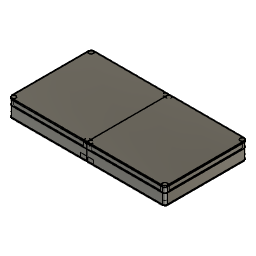
v1.3 (Autodesk Fusion 360 design; units mm, degrees)
Autodesk Fusion 360 part; units mm, degrees
(part 1 of 2)
sketch "Sketch1" plane through (0, 0, 0) normal (0, 0, 1) x (1, 0, 0)
  line L0 (192.147805, -6) -> (205.147805, -6) construction
  line L1 (192.147805, -6) -> (179.147805, -6) construction
  circle A0 centre (179.146093, -187.967124) radius 2
  circle A1 centre (13.147805, -188) radius 2
  line L2 (13.147805, -6) -> (13.147805, -16) construction
  circle A2 centre (205.147805, -16) radius 2
  line L3 (13.147805, -198) -> (13.147805, -188) construction
  line L4 (384.147805, -198) -> (371.147805, -198) construction
  line L5 (179.147805, -26) -> (13.147805, -26)
  line L6 (192.147805, -197.967124) -> (179.147805, -197.967124) construction
  line L7 (384.147805, -6) -> (371.147805, -6) construction
  line L8 (179.147805, -6) -> (179.147805, -26) construction
  line L9 (192.147805, -197.967124) -> (0.147805, -198)
  line L10 (205.147805, -197.967124) -> (205.147805, -187.967124) construction
  line L11 (0.147805, -198) -> (0.147805, -6)
  circle A3 centre (179.147805, -16) radius 2
  line L12 (384.147805, -198) -> (384.147805, -6)
  line L13 (371.147805, -26) -> (205.147805, -26)
  line L14 (371.147805, -198) -> (371.147805, -188) construction
  line L15 (205.147805, -26) -> (205.147805, -177.967124)
  line L16 (13.147805, -178) -> (179.147805, -178)
  line L17 (0.147805, -198) -> (13.147805, -198) construction
  line L18 (205.147805, -197.967124) -> (205.147805, -177.967124) construction
  circle A4 centre (205.147805, -187.967124) radius 2
  line L19 (0.147805, -198) -> (13.147805, -198) construction
  line L20 (371.147805, -6) -> (371.147805, -16) construction
  line L21 (192.147805, -6) -> (179.147805, -6) construction
  circle A5 centre (13.147805, -16) radius 2
  circle A6 centre (371.147805, -16) radius 2
  line L22 (192.147805, -6) -> (192.147805, -197.967124) construction
  line L23 (179.147805, -6) -> (179.147805, -16) construction
  line L24 (371.147805, -6) -> (371.147805, -26) construction
  line L25 (205.147805, -6) -> (205.147805, -16) construction
  line L26 (13.147805, -26) -> (13.147805, -178)
  line L27 (384.147805, -6) -> (0.147805, -6)
  line L28 (179.147805, -197.967124) -> (179.146093, -187.967124) construction
  line L29 (13.147805, -198) -> (13.147805, -178) construction
  line L30 (0.147805, -6) -> (13.147805, -6) construction
  line L31 (179.147805, -178) -> (179.147805, -26)
  line L32 (192.147805, -197.967124) -> (205.147805, -197.967124) construction
  line L33 (0.147805, -6) -> (0.147805, -198)
  line L34 (205.147805, -177.967124) -> (371.147805, -177.967124)
  circle A7 centre (371.147805, -188) radius 2
  line L35 (384.147805, -6) -> (371.147805, -6) construction
  line L36 (371.147805, -177.967124) -> (371.147805, -26)
  line L37 (0.147805, -198) -> (384.147805, -198)
  line L38 (192.147805, -197.967124) -> (205.147805, -197.967124) construction
  line L39 (384.147805, -6) -> (384.147805, 12.021307) construction
  line L40 (0.147805, -6) -> (-9.044583, 3.192388) construction
  line L41 (0.147805, -6) -> (15, -6) construction
  circle A8 centre (-4.448389, -1.403806) radius 6.5
  line L42 (0.147805, -198) -> (-9.044583, -207.192388) construction
  line L43 (384.147805, -198) -> (393.340193, -207.192388) construction
  line L44 (384.147805, -198) -> (399, -198) construction
  line L45 (384.147805, -6) -> (393.340193, 3.192388) construction
  line L46 (384.147805, -6) -> (399, -6) construction
  circle A9 centre (388.743999, -1.403806) radius 6.5
  circle A10 centre (388.743999, -202.596194) radius 6.5
  circle A11 centre (-4.448389, -202.596194) radius 6.5
  line L47 (-10.930518, -1.885465) -> (-10.948389, -202.595615)
  line L48 (-4.448389, -209.096194) -> (388.743999, -209.096194)
  line L49 (395.243999, -202.596194) -> (395.243999, -1.403806)
  line L50 (-4.448389, 5.096194) -> (388.743999, 5.096194)
  line L51 (388.743999, -202.596194) -> (395.243999, -202.596194) construction
  line L52 (-4.448389, -1.403806) -> (-4.448389, 5.096194) construction
  point P0 (13, -13)
  dimension "d13" = 192
  dimension "d14" = 192
  dimension "d15" = 384
  dimension "d16" = 384
  dimension "d20" = 13
  dimension "d21" = 10
  dimension "d22" = 4
  dimension "d23" = 13
  dimension "d24" = 10
  dimension "d25" = 13
  dimension "d26" = 10
  dimension "d27" = 13
  dimension "d28" = 10
  dimension "d29" = 13
  dimension "d30" = 10
  dimension "d31" = 13
  dimension "d32" = 10
  dimension "d33" = 13
  dimension "d34" = 10
  dimension "d35" = 13
  dimension "d36" = 10
  dimension "d37" = 4
  dimension "d38" = 4
  dimension "d39" = 4
  dimension "d40" = 4
  dimension "d41" = 4
  dimension "d42" = 4
  dimension "d43" = 4
  dimension "d44" = 13
  dimension "d45" = 20
  dimension "d46" = 13
  dimension "d47" = 20
  dimension "d48" = 13
  dimension "d49" = 20
  dimension "d50" = 13
  dimension "d51" = 20
  dimension "d69" = 135
  dimension "d70" = 13
  dimension "d71" = 13
  dimension "d72" = 45
  dimension "d73" = 13
  dimension "d74" = 13
  dimension "d75" = 45
  dimension "d104" = 135
  constraint perpendicular L11 L30
  constraint perpendicular L2 L30
  constraint perpendicular L7 L12
  constraint perpendicular L7 L20
  constraint perpendicular L4 L12
  constraint perpendicular L14 L37
  constraint perpendicular L19 L33
  constraint perpendicular L3 L19
  constraint perpendicular L22 L37
  constraint perpendicular L6 L22
  constraint perpendicular L9 L28
  constraint perpendicular L21 L22
  constraint perpendicular L21 L23
  constraint perpendicular L0 L22
  constraint perpendicular L25 L27
  constraint perpendicular L22 L32
  constraint perpendicular L10 L32
  constraint perpendicular L11 L17
  constraint perpendicular L17 L29
  constraint perpendicular L1 L22
  constraint perpendicular L1 L8
  constraint horizontal L16
  constraint vertical L31
  constraint horizontal L5
  constraint vertical L26
  constraint perpendicular L22 L38
  constraint perpendicular L18 L38
  constraint perpendicular L20 L35
  constraint perpendicular L24 L35
  constraint horizontal L34
  constraint vertical L36
  constraint horizontal L13
  constraint vertical L15
  constraint perpendicular L7 L39
  constraint horizontal L41
  constraint horizontal L44
  constraint horizontal L46
  constraint tangent A11 L47
  constraint tangent A10 L48
  constraint tangent A9 L49
  constraint perpendicular L46 L49
  constraint tangent A9 L50
  constraint perpendicular L49 L50
  constraint tangent A11 L48
  constraint parallel L48 L51
  constraint vertical L52
  measures "d22" diameter of A5
  measures "d37" diameter of A1
  measures "d38" diameter of A3
  measures "d39" diameter of A0
  measures "d40" diameter of A2
  measures "d41" diameter of A4
  measures "d42" diameter of A7
  measures "d43" diameter of A6
  measures "d69" angle of L40 L41
  measures "d72" angle of L43 L44
  measures "d75" angle of L45 L46
  measures "d104" angle of L37 L42
extrude "Extrude1" add sketch "Sketch1" along normal blind 2 contours L11 L33 A8 A11 L47 | L11 L12 L27 L33 L37 | L37 A10 A11 L48 | A11 | L27 A8 A9 L50 | A8 | L12 A9 A10 L49 | A10 | A9 picked at (-4.706637, -133.373076) picked at (187.814472, -127.322375) picked at (255.526246, -202.702251) picked at (-2.560006, -204.6862) picked at (255.526246, -1.297749) picked at (-3.056002, -1.357586) picked at (389.062427, -70.631992) picked at (386.660446, -202.382039) picked at (392.395412, 0.127516) makes body 1
sketch "Sketch3" plane through (0, 0, 2) normal (0, 0, 1) x (-1, 0, 0)
  arc A0 (-395.243999, 1.403816) -> (-388.743999, -5.096194) centre (-388.743999, 1.403806) ccw
  line L0 (-388.743999, -5.096194) -> (4.448389, -5.096194)
  arc A1 (4.448389, -5.096194) -> (10.930518, 1.885465) centre (4.448389, 1.403806) ccw
  circle A2 centre (4.448389, 1.403806) radius 5.5
  circle A3 centre (4.448389, 202.596194) radius 5.5
  circle A4 centre (-388.743999, 202.596194) radius 5.5
  circle A5 centre (-388.743999, 1.403806) radius 5.5
  line L1 (-388.743999, -4.096194) -> (4.448389, -4.096194)
  line L2 (9.948389, 1.403806) -> (9.948389, 202.596194)
  line L3 (3.313779, 207.977891) -> (-388.74234, 208.096194)
  line L4 (-394.243998, 202.59619) -> (-394.243999, 1.403806)
  line L5 (-192.147805, -4.096194) -> (-192.714281, 208.037042) construction
  circle A6 centre (-187.161139, 0.903806) radius 5
  circle A7 centre (-197.161175, 0.903806) radius 5
  circle A8 centre (-187.700907, 203.035529) radius 5
  circle A9 centre (-197.70095, 203.038547) radius 5
  line L6 (-182.700907, 203.035529) -> (-182.700907, 208.034021)
  line L7 (-202.700834, 203.072636) -> (-202.666966, 208.040046)
  line L8 (-187.161145, 5.903806) -> (-197.161175, 5.903806)
  line L9 (-202.161175, 0.903806) -> (-202.161175, -4.096194)
  line L10 (-182.161139, 0.903806) -> (-182.161139, -4.096194)
  line L11 (-383.661991, 197.999703) -> (-384.000006, 6)
  line L12 (0.338009, 197.999703) -> (-383.661991, 197.999703)
  line L13 (-0.000006, 6) -> (0.338009, 197.999703)
  line L14 (-384.000006, 6) -> (-0.000006, 6)
  line L15 (4.448389, 6.903806) -> (9.948389, 6.903806)
  line L16 (-1.051611, 1.403806) -> (-1.051611, -4.096194)
  line L17 (-383.243999, 1.403806) -> (-383.243999, -4.096194)
  line L18 (-388.743999, 6.903806) -> (-394.243999, 6.903806)
  line L19 (-388.743999, 197.096194) -> (-394.243998, 197.096194)
  line L20 (-383.243999, 202.596194) -> (-383.243999, 208.094535)
  line L21 (4.448389, 197.096194) -> (9.948389, 197.096194)
  line L22 (-1.051611, 202.596194) -> (-1.051611, 207.979208)
  circle A10 centre (-13.147805, 188) radius 2
  circle A11 centre (-179.146093, 187.967124) radius 2
  circle A12 centre (-205.147805, 16) radius 2
  circle A13 centre (-179.147805, 16) radius 2
  circle A14 centre (-205.147805, 187.967124) radius 2
  circle A15 centre (-13.147805, 16) radius 2
  circle A16 centre (-371.147805, 16) radius 2
  line L23 (-179.147805, 26) -> (-179.147805, 178)
  line L24 (-179.147805, 178) -> (-13.147805, 178)
  line L25 (-13.147805, 178) -> (-13.147805, 26)
  line L26 (-13.147805, 26) -> (-179.147805, 26)
  line L27 (-371.147805, 26) -> (-371.147805, 177.967124)
  line L28 (-371.147805, 177.967124) -> (-205.147805, 177.967124)
  line L29 (-205.147805, 177.967124) -> (-205.147805, 26)
  line L30 (-205.147805, 26) -> (-371.147805, 26)
  circle A17 centre (-371.147805, 188) radius 2
  line L31 (10.930518, 1.885465) -> (10.948389, 202.595615)
  arc A18 (10.948389, 202.595615) -> (4.448389, 209.096194) centre (4.448389, 202.596194) ccw
  line L32 (4.448389, 209.096194) -> (-388.743999, 209.096194)
  arc A19 (-388.743999, 209.096194) -> (-395.243999, 202.596194) centre (-388.743999, 202.596194) ccw
  line L33 (-395.243999, 202.596194) -> (-395.243999, 1.403816)
  line L34 (-187.700907, 198.035529) -> (-197.702459, 198.038547)
  dimension "d76" = 11
  dimension "d77" = 11
  dimension "d78" = 11
  dimension "d79" = 11
  dimension "d80" = 5
  dimension "d81" = 5
  dimension "d82" = 5
  dimension "d83" = 5
  dimension "d85" = 192
  dimension "d87" = 384
  constraint concentric A1 A2
  constraint concentric A0 A5
  constraint tangent A2 L1
  constraint parallel L0 L1
  constraint tangent A3 L2
  constraint tangent A4 L3
  constraint tangent A5 L4
  constraint tangent L1 A6
  constraint tangent L5 A6
  constraint tangent L5 A7
  constraint tangent L1 A7
  constraint tangent L5 A8
  constraint tangent L3 A8
  constraint tangent L5 A9
  constraint tangent L3 A9
  constraint tangent A8 L6
  constraint vertical L6
  constraint tangent A9 L7
  constraint tangent A7 L8
  constraint horizontal L8
  constraint tangent A7 L9
  constraint perpendicular L1 L9
  constraint tangent A6 L10
  constraint perpendicular L1 L10
  constraint tangent A2 L15
  constraint horizontal L15
  constraint tangent A2 L16
  constraint perpendicular L1 L16
  constraint tangent A5 L17
  constraint perpendicular L1 L17
  constraint tangent A5 L18
  constraint perpendicular L4 L18
  constraint tangent A4 L19
  constraint perpendicular L4 L19
  constraint tangent A4 L20
  constraint vertical L20
  constraint tangent A3 L21
  constraint horizontal L21
  constraint tangent A3 L22
  constraint vertical L22
  constraint tangent A9 L34
  measures "d76" diameter of A2
  measures "d77" diameter of A3
  measures "d78" diameter of A4
  measures "d79" diameter of A5
  measures "d80" radius of A6
  measures "d81" radius of A7
  measures "d82" radius of A8
  measures "d83" radius of A9
extrude "Extrude3" add sketch "Sketch3" along normal blind 10.5 contours A0 L0 A1 L31 A18 L32 A19 L33 | A2 | A2 L2 L15 | A8 A9 L34 | A2 L1 L16 | A3 L2 L21 | L1 A6 L10 | A3 | L1 A6 A7 | A6 | A3 L3 L22 | L1 A7 L9 | A7 | A6 A7 L8 | L3 A8 L6 | A5 L1 L17 | L3 A8 A9 | A8 | A5 | L3 A9 L7 | A9 | A5 L4 L18 | A4 L3 L20 | A4 L4 L19 | A4 picked at (-59.768043, 208.369808) picked at (4.871547, 2.733745) picked at (8.867841, 5.823258) picked at (-192.551057, 200.543091) picked at (0.028937, -3.015646) picked at (8.867841, 198.176742) picked at (-183.143455, -3.113878) picked at (6.016455, 204.38488) picked at (-192.311776, -1.590688) picked at (-188.337621, 1.772436) picked at (-0.062432, 206.883152) picked at (-201.178859, -3.113878) picked at (-198.420758, 1.99524) picked at (-192.311777, 3.3983) picked at (-183.68286, 207.052352) picked at (-384.324547, -3.015646) picked at (-192.549402, 205.532365) picked at (-186.168019, 202.106885) picked at (-390.721998, 2.844949) picked at (-201.698976, 207.06513) picked at (-199.037428, 203.173544) picked at (-393.163452, 5.823258) picked at (-384.324154, 207.014706) picked at (-393.16345, 198.176741) picked at (-387.470184, 206.100526) bodies 1
sketch "Sketch4" plane through (0, 0, 12.5) normal (0, 0, 1) x (-1, 0, 0)
  arc A0 (4.448389, -5.096194) -> (10.930518, 1.885465) centre (4.448389, 1.403806) ccw
  line L0 (-388.743999, -5.096194) -> (4.448389, -5.096194)
  circle A1 centre (4.448389, 1.403806) radius 5
  circle A2 centre (-187.161139, 0.903806) radius 5
  circle A3 centre (-197.161175, 0.903806) radius 5
  circle A4 centre (-388.743999, 1.403806) radius 5
  circle A5 centre (-388.743999, 202.596194) radius 5
  circle A6 centre (-197.70095, 203.038547) radius 5
  circle A7 centre (-187.700907, 203.035529) radius 5
  circle A8 centre (4.448389, 202.596194) radius 5
  line L1 (10.930518, 1.885465) -> (10.948389, 202.595615)
  arc A9 (10.948389, 202.595615) -> (4.448389, 209.096194) centre (4.448389, 202.596194) ccw
  line L2 (4.448389, 209.096194) -> (-388.743999, 209.096194)
  arc A10 (-388.743999, 209.096194) -> (-395.243999, 202.596194) centre (-388.743999, 202.596194) ccw
  line L3 (-395.243999, 202.596194) -> (-395.243999, 1.403816)
  arc A11 (-395.243999, 1.403816) -> (-388.743999, -5.096194) centre (-388.743999, 1.403806) ccw
  line L4 (-202.161175, -4.096194) -> (-383.243999, -4.096194)
  arc A12 (-383.243999, 1.403806) -> (-388.743999, 6.903806) centre (-388.743999, 1.403806) ccw
  line L5 (-394.243999, 6.903806) -> (-394.243998, 197.096194)
  arc A13 (-388.743999, 197.096194) -> (-383.243999, 202.596194) centre (-388.743999, 202.596194) ccw
  line L6 (-383.243999, 208.094535) -> (-202.666966, 208.040046)
  arc A14 (-1.051611, 202.596194) -> (4.448389, 197.096194) centre (4.448389, 202.596194) ccw
  line L7 (9.948389, 197.096194) -> (9.948389, 6.903806)
  arc A15 (4.448389, 6.903806) -> (-1.051611, 1.403806) centre (4.448389, 1.403806) ccw
  arc A16 (-187.700907, 198.035529) -> (-182.700907, 203.035529) centre (-187.700907, 203.035529) ccw
  line L8 (-182.700907, 203.035529) -> (-182.700907, 208.034021)
  line L9 (-182.700907, 208.034021) -> (-1.051611, 207.979208)
  line L10 (-1.051611, 207.979208) -> (-1.051611, 202.596194)
  line L11 (4.448389, 197.096194) -> (9.948389, 197.096194)
  line L12 (9.948389, 6.903806) -> (4.448389, 6.903806)
  line L13 (-1.051611, 1.403806) -> (-1.051611, -4.096194)
  line L14 (-1.051611, -4.096194) -> (-182.161139, -4.096194)
  line L15 (-182.161139, -4.096194) -> (-182.161139, 0.903806)
  arc A17 (-182.161139, 0.903806) -> (-187.161145, 5.903806) centre (-187.161139, 0.903806) ccw
  line L16 (-187.161145, 5.903806) -> (-197.161175, 5.903806)
  arc A18 (-197.161175, 5.903806) -> (-202.161175, 0.903806) centre (-197.161175, 0.903806) ccw
  line L17 (-202.161175, 0.903806) -> (-202.161175, -4.096194)
  line L18 (-394.243998, 197.096194) -> (-388.743999, 197.096194)
  line L19 (-383.243999, 202.596194) -> (-383.243999, 208.094535)
  line L20 (-202.666966, 208.040046) -> (-202.700834, 203.072636)
  arc A19 (-202.700834, 203.072636) -> (-197.702459, 198.038547) centre (-197.70095, 203.038547) ccw
  line L21 (-197.702459, 198.038547) -> (-187.700907, 198.035529)
  line L22 (-383.243999, -4.096194) -> (-383.243999, 1.403806)
  line L23 (-388.743999, 6.903806) -> (-394.243999, 6.903806)
  point P0 (3.978074, 2.11107)
  dimension "d90" = 10
  dimension "d91" = 10
  dimension "d92" = 10
  dimension "d93" = 10
  dimension "d94" = 10
  dimension "d95" = 10
  dimension "d96" = 10
  dimension "d97" = 10
  measures "d90" diameter of A1
  measures "d91" diameter of A2
  measures "d92" diameter of A3
  measures "d93" diameter of A4
  measures "d94" diameter of A5
  measures "d95" diameter of A6
  measures "d96" diameter of A7
  measures "d97" diameter of A8
extrude "Extrude4" cut sketch "Sketch4" against normal blind 3.2 contours A1 | A2 A17 | A3 A18 | A7 A16 | A6 A19 | A4 | A5 | A8 picked at (5.777141, 1.767992) picked at (-186.069705, 1.666582) picked at (-197.770077, -1.144458) picked at (-186.168019, 202.106885) picked at (-197.275592, 204.188268) picked at (-387.522246, 2.537427) picked at (-386.78051, 203.729815) picked at (6.023459, 204.03957) bodies 1
extrude "Extrude5" add 3 faces at (-9.918192, -4.172231, 12.5) (192.311777, -3.3983, 12.5) (192.551057, -200.543091, 12.5) along direction (0, 0, 1) blind 3 separate body on bodies 1 makes body 2
sketch "Sketch7" plane through (0, 0, 15.5) normal (0, 0, 1) x (-1, 0, 0)
  arc A0 (-197.702459, 198.038547) -> (-202.700834, 203.072636) centre (-197.70095, 203.038547) ccw
  line L0 (-197.702459, 198.038547) -> (-187.700907, 198.035529)
  arc A1 (-182.700907, 203.035529) -> (-187.700907, 198.035529) centre (-187.700907, 203.035529) ccw
  line L1 (-182.700907, 203.035529) -> (-182.700907, 208.034021)
  line L2 (-182.700907, 208.034021) -> (-1.051611, 207.979208)
  line L3 (-1.051611, 207.979208) -> (-1.051611, 202.596194)
  arc A2 (-1.051611, 202.596194) -> (4.448389, 197.096194) centre (4.448389, 202.596194) ccw
  line L4 (4.448389, 197.096194) -> (9.948389, 197.096194)
  line L5 (9.948389, 197.096194) -> (9.948389, 6.903806)
  line L6 (9.948389, 6.903806) -> (4.448389, 6.903806)
  arc A3 (4.448389, 6.903806) -> (-1.051611, 1.403806) centre (4.448389, 1.403806) ccw
  line L7 (-1.051611, 1.403806) -> (-1.051611, -4.096194)
  line L8 (-1.051611, -4.096194) -> (-182.161139, -4.096194)
  line L9 (-182.161139, -4.096194) -> (-182.161139, 0.903806)
  arc A4 (-187.161145, 5.903806) -> (-182.161139, 0.903806) centre (-187.161139, 0.903806) ccw
  line L10 (-187.161145, 5.903806) -> (-197.161175, 5.903806)
  arc A5 (-202.161175, 0.903806) -> (-197.161175, 5.903806) centre (-197.161175, 0.903806) ccw
  line L11 (-202.161175, 0.903806) -> (-202.161175, -4.096194)
  line L12 (-202.161175, -4.096194) -> (-383.243999, -4.096194)
  line L13 (-383.243999, -4.096194) -> (-383.243999, 1.403806)
  arc A6 (-383.243999, 1.403806) -> (-388.743999, 6.903806) centre (-388.743999, 1.403806) ccw
  line L14 (-388.743999, 6.903806) -> (-394.243999, 6.903806)
  line L15 (-394.243999, 6.903806) -> (-394.243998, 197.096194)
  line L16 (-394.243998, 197.096194) -> (-388.743999, 197.096194)
  arc A7 (-388.743999, 197.096194) -> (-383.243999, 202.596194) centre (-388.743999, 202.596194) ccw
  line L17 (-383.243999, 202.596194) -> (-383.243999, 208.094535)
  line L18 (-383.243999, 208.094535) -> (-202.666966, 208.040046)
  line L19 (-202.666966, 208.040046) -> (-202.700834, 203.072636)
  circle A8 centre (-388.743999, 202.596194) radius 5
  circle A9 centre (4.448389, 1.403806) radius 5
  circle A10 centre (-388.743999, 1.403806) radius 5
  circle A11 centre (4.448389, 202.596194) radius 5
  line L20 (-395.243999, 202.596194) -> (-395.243999, 1.403816)
  arc A12 (-395.243999, 1.403816) -> (-388.743999, -5.096194) centre (-388.743999, 1.403806) ccw
  line L21 (-388.743999, -5.096194) -> (4.448389, -5.096194)
  arc A13 (4.448389, -5.096194) -> (10.930518, 1.885465) centre (4.448389, 1.403806) ccw
  line L22 (10.930518, 1.885465) -> (10.948389, 202.595615)
  arc A14 (10.948389, 202.595615) -> (4.448389, 209.096194) centre (4.448389, 202.596194) ccw
  line L23 (4.448389, 209.096194) -> (-388.743999, 209.096194)
  arc A15 (-388.743999, 209.096194) -> (-395.243999, 202.596194) centre (-388.743999, 202.596194) ccw
  circle A16 centre (4.448389, 202.596194) radius 6.5
  circle A17 centre (4.448389, 1.403806) radius 6.5
  circle A18 centre (-388.743999, 1.403806) radius 6.5
  circle A19 centre (-388.743999, 202.596194) radius 6.5
  spline S0 degree 5 poles (10.946693, 1.25535) (10.946761, 9.30896) (10.946897, 25.416182) (10.9471, 49.577014) (10.947372, 81.791456) (10.947711, 122.059509) (10.947982, 154.273952) (10.948185, 178.434783) (10.948321, 194.542005) (10.948389, 202.595615) knots 0 0 0 0 0 0 0.2 0.4 0.6 0.8 1 1 1 1 1 1
  line L24 (4.448389, 209.096194) -> (-388.743999, 209.096194)
  line L25 (-395.243999, 202.596194) -> (-395.243999, 1.403816)
  line L26 (-388.743999, -5.096194) -> (4.448389, -5.096194)
  constraint concentric A2 A16
  constraint concentric A3 A17
  constraint concentric A6 A18
  constraint concentric A7 A19
extrude "Extrude7" add sketch "Sketch7" along normal blind 0.5 contours A4 L10 A5 | A0 A1 L1 L2 L3 L4 L5 L6 L7 L8 L9 A4 A5 L11 L12 L13 L14 L15 L16 L17 L18 L19 A16 A17 A18 A19 | A0 A1 L1 L2 L3 L17 L18 L19 L23 A16 A19 L24 | A0 L0 A1 | L16 A7 L17 A19 | L16 A7 L17 A15 A19 | L3 A2 L4 A14 A16 | L3 A2 L4 A16 | L4 L5 L6 L22 A16 A17 S0 | L14 L15 L16 L20 A18 A19 L25 | L13 A6 L14 A12 A18 | L6 A3 L7 A13 A17 S0 | L7 L8 L9 A4 A5 L11 L12 L13 L21 A17 A18 L26 | L13 A6 L14 A18 | L6 A3 L7 A17 | A8 | A9 | A10 | A11 picked at (-192.311777, 3.3983) picked at (-125.003286, 133.979778) picked at (-324.573843, 208.387801) picked at (-192.550905, 200.54222) picked at (-389.022173, 196.449435) picked at (-383.484711, 204.242153) picked at (-0.810899, 204.242153) picked at (0.429343, 197.93514) picked at (10.259265, 135.220919) picked at (-394.554875, 135.220919) picked at (-383.484711, -0.242153) picked at (-0.810899, -0.242153) picked at (-190.485583, -4.762861) picked at (-389.022173, 7.550565) picked at (0.429343, 6.06486) picked at (-386.78051, 203.729815) picked at (5.825453, 2.342673) picked at (-387.522246, 2.537427) picked at (3.831203, 204.2582) bodies 2
sketch "Sketch8" plane through (0, 0, 2) normal (0, 0, 1) x (-1, 0, 0)
  line L0 (-197.161175, 5.903806) -> (-187.161145, 5.903806)
  arc A0 (-182.161139, 0.903806) -> (-187.161145, 5.903806) centre (-187.161139, 0.903806) ccw
  line L1 (-182.161139, 0.903806) -> (-182.161139, -4.096194)
  line L2 (-182.161139, -4.096194) -> (-1.051611, -4.096194)
  line L3 (-1.051611, -4.096194) -> (-1.051611, 1.403806)
  arc A1 (4.448389, 6.903806) -> (-1.051611, 1.403806) centre (4.448389, 1.403806) ccw
  line L4 (4.448389, 6.903806) -> (9.948389, 6.903806)
  line L5 (9.948389, 6.903806) -> (9.948389, 197.096194)
  line L6 (9.948389, 197.096194) -> (4.448389, 197.096194)
  arc A2 (-1.051611, 202.596194) -> (4.448389, 197.096194) centre (4.448389, 202.596194) ccw
  line L7 (-1.051611, 202.596194) -> (-1.051611, 207.979208)
  line L8 (-1.051611, 207.979208) -> (-182.700907, 208.034021)
  line L9 (-182.700907, 208.034021) -> (-182.700907, 203.035529)
  arc A3 (-187.700907, 198.035529) -> (-182.700907, 203.035529) centre (-187.700907, 203.035529) ccw
  line L10 (-187.700907, 198.035529) -> (-197.702459, 198.038547)
  circle A4 centre (-179.147805, 16) radius 2
  circle A5 centre (-13.147805, 16) radius 2
  line L11 (-179.147805, 26) -> (-179.147805, 178)
  line L12 (-179.147805, 178) -> (-13.147805, 178)
  line L13 (-13.147805, 178) -> (-13.147805, 26)
  line L14 (-13.147805, 26) -> (-179.147805, 26)
  circle A6 centre (-13.147805, 188) radius 2
  circle A7 centre (-179.146093, 187.967124) radius 2
  line L15 (-13.147805, 102) -> (-179.147805, 102) construction
  line L16 (-96.147805, 26) -> (-96.147805, 178) construction
  line L17 (-96.147805, 26) -> (-96.147805, -4.096194) construction
  line L18 (-13.147805, 102) -> (9.948389, 102) construction
  line L19 (-179.147805, 102) -> (-179.152649, 101.99983) construction
  line L20 (-179.152649, 101.99983) -> (-194.251759, 101.99983) construction
  line L21 (-96.147805, 178) -> (-96.13875, 208.007901) construction
  circle A8 centre (-96.147805, 10.951903) radius 4
  circle A9 centre (-1.599708, 102) radius 4
  circle A10 centre (-186.702204, 101.99983) radius 4
  circle A11 centre (-96.143278, 193.00395) radius 4
  circle A12 centre (-288.16487, 10.960451) radius 4
  circle A13 centre (-382.70486, 102.016966) radius 4
  circle A14 centre (-288.153189, 193.012498) radius 4
  circle A15 centre (-198.232599, 101.97088) radius 4
  line L22 (-194.296332, 43.951818) -> (-190.296332, 43.951818)
  line L23 (-190.296332, 43.951818) -> (-190.296332, 63.951818)
  line L24 (-190.296332, 63.951818) -> (-194.296332, 63.951818)
  line L25 (-194.296332, 63.951818) -> (-194.296332, 43.951818)
  line L26 (-194.296332, 43.951818) -> (-190.296332, 63.951818) construction
  line L27 (-190.296332, 43.951818) -> (-194.296332, 63.951818) construction
  line L28 (-190.566594, 160.018434) -> (-194.566594, 160.018434)
  line L29 (-194.566594, 160.018434) -> (-194.566594, 140.018434)
  line L30 (-194.566594, 140.018434) -> (-190.566594, 140.018434)
  line L31 (-190.566594, 140.018434) -> (-190.566594, 160.018434)
  line L32 (-190.566594, 160.018434) -> (-194.566594, 140.018434) construction
  line L33 (-194.566594, 160.018434) -> (-190.566594, 140.018434) construction
  arc A16 (-202.700834, 203.072636) -> (-197.702459, 198.038547) centre (-197.70095, 203.038547) ccw
  line L34 (-202.700834, 203.072636) -> (-202.666966, 208.040046)
  line L35 (-202.666966, 208.040046) -> (-383.243999, 208.094535)
  line L36 (-383.243999, 208.094535) -> (-383.243999, 202.596194)
  arc A17 (-388.743999, 197.096194) -> (-383.243999, 202.596194) centre (-388.743999, 202.596194) ccw
  line L37 (-388.743999, 197.096194) -> (-394.243998, 197.096194)
  line L38 (-394.243998, 197.096194) -> (-394.243999, 6.903806)
  line L39 (-394.243999, 6.903806) -> (-388.743999, 6.903806)
  arc A18 (-383.243999, 1.403806) -> (-388.743999, 6.903806) centre (-388.743999, 1.403806) ccw
  line L40 (-383.243999, 1.403806) -> (-383.243999, -4.096194)
  line L41 (-383.243999, -4.096194) -> (-202.161175, -4.096194)
  line L42 (-202.161175, -4.096194) -> (-202.161175, 0.903806)
  arc A19 (-197.161175, 5.903806) -> (-202.161175, 0.903806) centre (-197.161175, 0.903806) ccw
  circle A20 centre (-205.147805, 16) radius 2
  circle A21 centre (-205.147805, 187.967124) radius 2
  circle A22 centre (-371.147805, 16) radius 2
  line L43 (-371.147805, 26) -> (-371.147805, 177.967124)
  line L44 (-371.147805, 177.967124) -> (-205.147805, 177.967124)
  line L45 (-205.147805, 177.967124) -> (-205.147805, 26)
  line L46 (-205.147805, 26) -> (-371.147805, 26)
  circle A23 centre (-371.147805, 188) radius 2
  line L47 (-192.701683, 198.037038) -> (-192.431504, 101.99983) construction
  line L48 (-192.431504, 101.99983) -> (-192.16116, 5.903806) construction
  line L49 (-179.152649, 101.99983) -> (-190.702197, 101.992602)
  line L50 (-192.431481, 101.99152) -> (-205.147805, 101.983562)
  line L51 (-190.702197, 101.992602) -> (-192.431481, 101.99152)
  point P0 (-192.296332, 53.951818)
  point P1 (-192.566594, 150.018434)
  dimension "d107" = 8
  dimension "d108" = 8
  dimension "d109" = 8
  dimension "d110" = 8
  dimension "d119" = 4
  dimension "d120" = 20
  dimension "d121" = 4
  dimension "d122" = 20
  constraint perpendicular L2 L17
  constraint horizontal L20
  constraint perpendicular L8 L21
  constraint horizontal L22
  constraint perpendicular L22 L23
  constraint parallel L22 L24
  constraint parallel L23 L25
  constraint horizontal L28
  constraint perpendicular L28 L29
  constraint parallel L28 L30
  constraint parallel L29 L31
  measures "d107" diameter of A8
  measures "d108" diameter of A9
  measures "d109" diameter of A10
  measures "d110" diameter of A11
extrude "Extrude8" cut sketch "Sketch8" against normal blind 1 contours A8 | A9 | A10 L49 | A10 L49 | A11 | A12 | A13 | A14 | A15 L50 | A15 L50 picked at (-93.851962, 12.057523) picked at (-2.964592, 101.181543) picked at (-187.297966, 104.597667) picked at (-186.446413, 100.005214) picked at (-94.809944, 191.846927) picked at (-288.479546, 8.575186) picked at (-381.865748, 99.718165) picked at (-286.879092, 190.805697) picked at (-198.771809, 100.245188) picked at (-197.469271, 104.463151) bodies 1
ref_plane "WorkPlane3" through (192.152272, -102.254102, 6.25) normal (-1, 0.00004452, 0) x (-0.00004452, -1, 0)
sketch "Sketch9" plane through (0, 0, 1) normal (0, 0, 1) x (-1, 0, 0)
  circle A0 centre (-96.147805, 10.951903) radius 4
  circle A1 centre (-96.147805, 10.951903) radius 2
  circle A2 centre (-96.149998, 192.999996) radius 4.000312 construction
  circle A3 centre (-186.071543, 101.964847) radius 3.997635 construction
  circle A4 centre (-1.596451, 102.000736) radius 3.997495 construction
  circle A5 centre (-1.596451, 102.000736) radius 2
  circle A6 centre (-96.149998, 192.999996) radius 2
  circle A7 centre (-186.071543, 101.964847) radius 2
  line L0 (-192.146912, 222.691031) -> (-192.157647, -18.450486)
  circle A8 centre (-382.708118, 102.017702) radius 2
  circle A9 centre (-288.146469, 193.008543) radius 2
  circle A10 centre (-198.233029, 101.965388) radius 2
  circle A11 centre (-288.16487, 10.960451) radius 2
  point P0 (-382.708118, 102.017702)
  dimension "d113" = 4
  dimension "d114" = 4
  dimension "d115" = 4
  dimension "d116" = 4
  constraint concentric A0 A1
  constraint concentric A4 A5
  constraint concentric A2 A6
  constraint concentric A3 A7
  constraint symmetric A1 L0 A11
  constraint symmetric A5 L0 A8
  constraint symmetric A6 L0 A9
  constraint symmetric A7 L0 A10
  measures "d113" diameter of A1
  measures "d114" diameter of A5
  measures "d115" diameter of A6
  measures "d116" diameter of A7
extrude "Extrude9" cut sketch "Sketch9" against normal blind 1 contours A1 | A5 | A6 | A7 | A8 | A9 | A10 | A11 picked at (-96.933201, 10.498454) picked at (-1.085577, 101.251423) picked at (-95.816665, 193.776069) picked at (-185.434495, 100.861446) picked at (-383.367338, 102.117064) picked at (-288.805689, 192.909181) picked at (-197.595981, 100.861988) picked at (-287.50565, 10.86109) bodies 1
split "Split3" by plane through (192.152272, -102.254102, 6.25) normal (-1, 0.00004452, 0) bodies 2 1 makes body 4 at (0.834672, -42.791567, 0) makes body 3 at (124.458016, -68.628488, 16)
sketch "Sketch13" plane through (0, 0, 0) normal (0, 0, -1) x (1, 0, 0)
  line L0 (192.157051, -5.096194) -> (192.147516, 209.096194)
  line L1 (192.147516, 209.096194) -> (-4.448389, 209.096194)
  arc A0 (-4.448389, 209.096194) -> (-10.948389, 202.595615) centre (-4.448389, 202.596194) ccw
  line L2 (-10.948389, 202.595615) -> (-10.930518, 1.885465)
  arc A1 (-10.930518, 1.885465) -> (-4.448389, -5.096194) centre (-4.448389, 1.403806) ccw
  line L3 (-4.448389, -5.096194) -> (192.157051, -5.096194)
  circle A2 centre (13.147805, 188) radius 2
  line L4 (179.147805, 178) -> (179.147805, 26)
  line L5 (179.147805, 26) -> (13.147805, 26)
  line L6 (13.147805, 26) -> (13.147805, 178)
  line L7 (13.147805, 178) -> (179.147805, 178)
  circle A3 centre (13.147805, 16) radius 2
  circle A4 centre (179.147805, 16) radius 2
  circle A5 centre (1.596451, 102.000736) radius 2
  circle A6 centre (96.147805, 10.951903) radius 2
  circle A7 centre (96.149998, 192.999996) radius 2
  circle A8 centre (186.071543, 101.964847) radius 2
  line L8 (192.147805, 6.032876) -> (205.147805, 6.032876) construction
  circle A9 centre (371.147805, 188) radius 2
  line L9 (384.147805, 6) -> (399, 6) construction
  line L10 (371.147805, 26.032876) -> (371.147805, 178)
  line L11 (384.147805, 198) -> (399, 198) construction
  line L12 (384.147805, 198) -> (371.147805, 198) construction
  line L13 (192.147805, 6.032876) -> (205.147805, 6.032876) construction
  line L14 (395.243999, 1.403806) -> (395.243999, 202.596194)
  line L15 (388.743999, 1.403806) -> (395.243999, 1.403806) construction
  line L16 (371.147805, 178) -> (205.147805, 178)
  line L17 (371.147805, 6) -> (371.147805, 16) construction
  line L18 (0.147805, 198) -> (15, 198) construction
  line L19 (384.147805, 6) -> (371.147805, 6) construction
  line L20 (-4.448389, -5.096194) -> (388.743999, -5.096194)
  line L21 (384.147805, 198) -> (0.147805, 198)
  line L22 (205.147805, 178) -> (205.147805, 26.032876)
  line L23 (205.147805, 6.032876) -> (205.147805, 16.032876) construction
  line L24 (371.147805, 198) -> (371.147805, 188) construction
  line L25 (384.147805, 198) -> (384.147805, 216.021307) construction
  circle A10 centre (388.743999, 202.596194) radius 6.5
  line L26 (179.147805, 198) -> (179.147805, 178) construction
  line L27 (0.147805, 6) -> (0.147805, 198)
  line L28 (179.147805, 6.032876) -> (179.146093, 16.032876) construction
  line L29 (384.147805, 198) -> (393.340193, 207.192388) construction
  line L30 (205.147805, 198) -> (205.147805, 188) construction
  circle A11 centre (388.743999, 1.403806) radius 6.5
  line L31 (-4.448389, 209.096194) -> (388.743999, 209.096194)
  line L32 (192.147805, 6.032876) -> (0.147805, 6)
  line L33 (13.147805, 198) -> (13.147805, 188) construction
  line L34 (13.147805, 178) -> (13.147805, 26)
  line L35 (179.147805, 198) -> (179.147805, 188) construction
  line L36 (13.147805, 6) -> (13.147805, 26) construction
  line L37 (192.147805, 198) -> (179.147805, 198) construction
  line L38 (0.147805, 6) -> (13.147805, 6) construction
  line L39 (0.147805, 6) -> (-9.044583, -3.192388) construction
  line L40 (-10.930518, 202.114535) -> (-10.948389, 1.404385)
  line L41 (179.147805, 178) -> (13.147805, 178)
  line L42 (13.147805, 6) -> (13.147805, 16) construction
  line L43 (0.147805, 198) -> (-9.044583, 207.192388) construction
  line L44 (-4.448389, 202.596194) -> (-4.448389, 209.096194) construction
  line L45 (0.147805, 198) -> (13.147805, 198) construction
  circle A12 centre (-4.448389, 202.596194) radius 6.5
  line L46 (0.147805, 198) -> (0.147805, 6)
  line L47 (13.147805, 26) -> (179.147805, 26)
  circle A13 centre (-4.448389, 1.403806) radius 6.5
  line L48 (192.147805, 198) -> (179.147805, 198) construction
  line L49 (0.147805, 6) -> (13.147805, 6) construction
  line L50 (192.147805, 198) -> (192.147805, 6.032876) construction
  line L51 (192.147805, 6.032876) -> (179.147805, 6.032876) construction
  line L52 (179.147805, 26) -> (179.147805, 178)
  line L53 (371.147805, 198) -> (371.147805, 178) construction
  line L54 (384.147805, 198) -> (371.147805, 198) construction
  line L55 (205.147805, 26.032876) -> (371.147805, 26.032876)
  line L56 (205.147805, 6.032876) -> (205.147805, 26.032876) construction
  line L57 (0.147805, 6) -> (384.147805, 6)
  line L58 (192.147805, 198) -> (205.147805, 198) construction
  line L59 (384.147805, 6) -> (393.340193, -3.192388) construction
  line L60 (384.147805, 6) -> (384.147805, 198)
  line L61 (13.147805, 178) -> (179.147805, 178)
  line L62 (179.147805, 178) -> (179.147805, 26)
  line L63 (179.147805, 26) -> (13.147805, 26)
  line L64 (13.147805, 26) -> (13.147805, 178)
  line L65 (205.147805, 26.032876) -> (371.147805, 26.032876)
  line L66 (371.147805, 26.032876) -> (371.147805, 178)
  line L67 (371.147805, 178) -> (205.147805, 178)
  line L68 (205.147805, 178) -> (205.147805, 26.032876)
  circle A14 centre (96.149998, 192.999996) radius 2
  circle A15 centre (186.071543, 101.964847) radius 2
  circle A16 centre (96.147805, 10.951903) radius 2
  circle A17 centre (1.596451, 102.000736) radius 2
  circle A18 centre (288.145613, 192.999996) radius 2
  circle A19 centre (382.69916, 102.000736) radius 2
  circle A20 centre (288.147805, 10.951903) radius 2
  circle A21 centre (198.224067, 101.964847) radius 2
  point P0 (13, 191)
  point P1 (0, 204)
  point P2 (288.147805, 10.951903)
  point P3 (198.224067, 101.964847)
  dimension "d136" = 192
  dimension "d137" = 192
  dimension "d138" = 384
  dimension "d139" = 384
  dimension "d140" = 13
  dimension "d141" = 10
  dimension "d143" = 13
  dimension "d144" = 10
  dimension "d145" = 13
  dimension "d146" = 10
  dimension "d147" = 13
  dimension "d148" = 10
  dimension "d149" = 13
  dimension "d150" = 10
  dimension "d151" = 13
  dimension "d152" = 10
  dimension "d153" = 13
  dimension "d154" = 10
  dimension "d155" = 13
  dimension "d156" = 10
  dimension "d163" = 4
  dimension "d164" = 13
  dimension "d165" = 20
  dimension "d166" = 13
  dimension "d167" = 20
  dimension "d168" = 13
  dimension "d169" = 20
  dimension "d170" = 13
  dimension "d171" = 20
  dimension "d172" = 135
  dimension "d173" = 13
  dimension "d174" = 13
  dimension "d175" = 45
  dimension "d176" = 13
  dimension "d177" = 13
  dimension "d178" = 45
  dimension "d179" = 135
  constraint perpendicular L27 L45
  constraint perpendicular L33 L45
  constraint perpendicular L12 L60
  constraint perpendicular L12 L24
  constraint perpendicular L19 L60
  constraint perpendicular L17 L57
  constraint perpendicular L38 L46
  constraint perpendicular L38 L42
  constraint perpendicular L50 L57
  constraint perpendicular L50 L51
  constraint perpendicular L28 L32
  constraint perpendicular L37 L50
  constraint perpendicular L35 L37
  constraint perpendicular L50 L58
  constraint perpendicular L21 L30
  constraint perpendicular L8 L50
  constraint perpendicular L8 L23
  constraint perpendicular L27 L49
  constraint perpendicular L36 L49
  constraint perpendicular L48 L50
  constraint perpendicular L26 L48
  constraint horizontal L47
  constraint vertical L52
  constraint horizontal L41
  constraint vertical L34
  constraint perpendicular L13 L50
  constraint perpendicular L13 L56
  constraint perpendicular L24 L54
  constraint perpendicular L53 L54
  constraint horizontal L55
  constraint vertical L10
  constraint horizontal L16
  constraint vertical L22
  constraint perpendicular L12 L25
  constraint horizontal L18
  constraint horizontal L9
  constraint horizontal L11
  constraint tangent L40 A13
  constraint tangent L20 A11
  constraint tangent L14 A10
  constraint perpendicular L11 L14
  constraint tangent A10 L31
  constraint perpendicular L14 L31
  constraint tangent L20 A13
  constraint parallel L15 L20
  constraint vertical L44
  constraint horizontal L61
  constraint vertical L62
  constraint horizontal L63
  constraint vertical L64
  constraint horizontal L65
  constraint vertical L66
  constraint horizontal L67
  constraint vertical L68
  constraint concentric A7 A14
  constraint concentric A8 A15
  constraint concentric A6 A16
  constraint concentric A5 A17
  constraint symmetric L50 A14 A18
  constraint symmetric L50 A17 A19
  constraint symmetric L50 A16 A20
  constraint symmetric L50 A15 A21
  measures "d163" diameter of A9
  measures "d172" angle of L18 L43
  measures "d175" angle of L9 L59
  measures "d178" angle of L11 L29
  measures "d179" angle of L39 L57
extrude "Extrude15" add sketch "Sketch13" 1 faces at (383.532315, -42.698421, 0) along normal blind 2 separate body contours L0 L3 L20 A13 L57 | L0 A5 L21 L27 L46 L57 A17 | L0 L21 L57 L60 A19 | A1 A13 | L0 L1 L21 L31 A12 | L0 L21 A10 L31 | L2 A5 L27 L40 A12 L46 A13 A17 | L14 A10 A11 L60 A19 | A10 | A0 A12 | A2 | A3 | A4 | A9 picked at (128.788406, 0.769204) picked at (156.392621, 189.999999) picked at (348.391822, 13.994926) picked at (-6.032309, -0.102931) picked at (128.782379, 203.230796) picked at (255.515785, 203.124483) picked at (-5.232329, 70.169846) picked at (391.313006, 102.000245) picked at (386.867376, 204.306189) picked at (-2.591007, 200.515121) picked at (13.563465, 188.719944) picked at (13.720803, 15.527311) picked at (178.990467, 14.807367) picked at (370.488585, 187.900638) on bodies 1 makes body 5
sketch "Sketch14" plane through (0, 0, -2) normal (0, 0, -1) x (1, 0, 0)
  line L0 (205.147805, 26.032876) -> (205.147805, 177.967124)
  line L1 (205.147805, 177.967124) -> (371.147805, 177.967124)
  line L2 (371.147805, 177.967124) -> (371.147805, 26.032876)
  line L3 (371.147805, 26.032876) -> (205.147805, 26.032876)
  arc A0 (380.935047, 102.943024) -> (384.47223, 101.075414) centre (382.708118, 102.017702) ccw
  arc A1 (384.47223, 101.075414) -> (380.935047, 102.943024) centre (382.69916, 102.000736) ccw
  arc A2 (198.107947, 103.961473) -> (198.34915, 99.968762) centre (198.233029, 101.965388) ccw
  arc A3 (198.34915, 99.968762) -> (198.107947, 103.961473) centre (198.224067, 101.964847) ccw
  circle A4 centre (186.071543, 101.964847) radius 2
  circle A5 centre (1.596451, 102.000736) radius 2
  line L4 (179.147805, 26) -> (13.147805, 26)
  line L5 (13.147805, 26) -> (13.147805, 178)
  line L6 (13.147805, 178) -> (179.147805, 178)
  line L7 (179.147805, 178) -> (179.147805, 26)
  circle A6 centre (96.149998, 192.999996) radius 2
  circle A7 centre (96.147805, 10.951903) radius 2
  line L8 (388.743999, 209.096194) -> (-4.448389, 209.096194)
  arc A8 (-4.448389, 209.096194) -> (-10.930518, 202.114535) centre (-4.448389, 202.596194) ccw
  line L9 (-10.930518, 202.114535) -> (-10.939432, 102)
  line L10 (-10.939432, 102) -> (-10.930518, 1.885465)
  arc A9 (-10.930518, 1.885465) -> (-4.448389, -5.096194) centre (-4.448389, 1.403806) ccw
  line L11 (-4.448389, -5.096194) -> (388.743999, -5.096194)
  arc A10 (388.743999, -5.096194) -> (395.243999, 1.403816) centre (388.743999, 1.403806) ccw
  line L12 (395.243999, 1.403806) -> (395.243999, 202.596194)
  arc A11 (395.243999, 202.596194) -> (388.743999, 209.096194) centre (388.743999, 202.596194) ccw
  arc A12 (286.156007, 193.203633) -> (290.136075, 192.804906) centre (288.146469, 193.008543) ccw
  arc A13 (290.136075, 192.804906) -> (286.156007, 193.203633) centre (288.145613, 192.999996) ccw
  arc A14 (287.260608, 12.744354) -> (289.052067, 9.168) centre (288.16487, 10.960451) ccw
  arc A15 (289.052067, 9.168) -> (287.260608, 12.744354) centre (288.147805, 10.951903) ccw
  line L13 (192.147805, 102) -> (192.147805, -5.096194) construction
  line L14 (192.147805, 102) -> (205.147805, 102) construction
  line L15 (192.147805, 102) -> (179.147805, 102) construction
  line L16 (192.147805, 209.096194) -> (192.147805, 102) construction
  line L17 (190.147805, 175.548097) -> (194.147805, 175.548097)
  line L18 (194.147805, 175.548097) -> (194.147805, 135.548097)
  line L19 (194.147805, 135.548097) -> (190.147805, 135.548097)
  line L20 (190.147805, 135.548097) -> (190.147805, 175.548097)
  line L21 (190.147805, 175.548097) -> (194.147805, 135.548097) construction
  line L22 (194.147805, 175.548097) -> (190.147805, 135.548097) construction
  line L23 (194.147805, 68.451903) -> (190.147805, 68.451903)
  line L24 (190.147805, 68.451903) -> (190.147805, 28.451903)
  line L25 (190.147805, 28.451903) -> (194.147805, 28.451903)
  line L26 (194.147805, 28.451903) -> (194.147805, 68.451903)
  line L27 (194.147805, 68.451903) -> (190.147805, 28.451903) construction
  line L28 (190.147805, 68.451903) -> (194.147805, 28.451903) construction
  line L29 (96.147805, 10.951903) -> (-10.931325, 10.942369) construction
  line L30 (96.147805, 10.951903) -> (192.147805, 10.951903) construction
  line L31 (13.147805, 26) -> (13.149146, 10.944513) construction
  circle A16 centre (13.149146, 10.944513) radius 2.5
  line L32 (13.149146, 10.944513) -> (71.149146, 10.944513) construction
  circle A17 centre (71.149146, 10.944513) radius 2.5
  line L33 (13.149146, 10.944513) -> (13.149146, 59.944513) construction
  circle A18 centre (13.149146, 59.944513) radius 2.5
  line L34 (71.149146, 10.944513) -> (71.144783, 59.944513) construction
  circle A19 centre (71.144783, 59.944513) radius 2.5
  line L35 (13.147805, 62.444513) -> (71.144783, 62.444513)
  line L36 (73.64914, 10.9499) -> (73.644783, 59.944735)
  circle A20 centre (13.149146, 59.944513) radius 1.5
  circle A21 centre (71.144783, 59.944513) radius 1.5
  circle A22 centre (71.149146, 10.944513) radius 1.5
  circle A23 centre (13.149146, 10.944513) radius 1.5
  point P0 (192.147805, 155.548097)
  point P1 (192.147805, 48.451903)
  dimension "d182" = 4
  dimension "d183" = 40
  dimension "d184" = 4
  dimension "d185" = 40
  dimension "d186" = 5
  dimension "d187" = 58
  dimension "d188" = 5
  dimension "d189" = 49
  dimension "d190" = 5
  dimension "d191" = 49
  dimension "d192" = 5
  dimension "d193" = 3
  dimension "d194" = 3
  dimension "d195" = 3
  dimension "d196" = 3
  constraint horizontal L17
  constraint perpendicular L17 L18
  constraint parallel L17 L19
  constraint parallel L18 L20
  constraint horizontal L23
  constraint perpendicular L23 L24
  constraint parallel L23 L25
  constraint parallel L24 L26
  constraint perpendicular L10 L29
  constraint perpendicular L13 L30
  constraint perpendicular L29 L31
  constraint perpendicular L7 L32
  constraint perpendicular L32 L33
  constraint perpendicular L29 L34
  constraint tangent A19 L35
  constraint tangent A19 L36
  constraint concentric A17 A22
  measures "d186" diameter of A16
  measures "d188" diameter of A17
  measures "d190" diameter of A18
  measures "d192" diameter of A19
  measures "d193" diameter of A20
  measures "d194" diameter of A21
  measures "d195" diameter of A22
  measures "d196" diameter of A23
extrude "Extrude16" add sketch "Sketch14" against normal blind 2 contours L4 L5 A18 A19 L35 L36 | A19 | L5 A18 A20 | L5 A20 | A22 | A23 picked at (51.977457, 36.818422) picked at (70.985142, 62.100762) picked at (13.337648, 62.097724) picked at (12.807994, 59.578146) picked at (70.61488, 11.335429) picked at (13.324416, 11.377526) bodies 5
extrude "Extrude17" add sketch "Sketch14" along normal blind 2 contours A19 | L5 A18 A20 | L5 A18 A20 | A16 | A17 picked at (70.985142, 62.100762) picked at (13.02365, 57.787215) picked at (13.337648, 62.097724) picked at (15.30092, 10.74579) picked at (73.300655, 11.146765) bodies 5
extrude "Extrude18" cut sketch "Sketch14" against normal blind 2 contours L5 A20 | A22 | A23 picked at (12.807994, 59.578146) picked at (70.61488, 11.335429) picked at (13.324416, 11.377526) bodies 5
extrude "Extrude19" add sketch "Sketch14" along normal blind 15 contours L17 L18 L19 L20 | L23 L24 L25 L26 picked at (192.814472, 162.214764) picked at (191.481139, 41.785236) bodies 5
sketch "Sketch15" plane through (190.147805, 0, 0) normal (-1, 0, 0) x (0, -1, 0)
  line L0 (175.548097, -2) -> (135.548097, -2)
  line L1 (135.548097, -2) -> (135.548097, -17)
  line L2 (135.548097, -17) -> (175.548097, -17)
  line L3 (175.548097, -17) -> (175.548097, -2)
  line L4 (155.548097, -17) -> (155.548097, -2) construction
  line L5 (135.548097, -2) -> (155.548097, -17) construction
  line L6 (155.548097, -17) -> (175.548097, -2) construction
  circle A0 centre (165.548097, -9.5) radius 2
  circle A1 centre (145.548097, -9.5) radius 2
  dimension "d205" = 4
  dimension "d206" = 4
  measures "d205" diameter of A0
  measures "d206" diameter of A1
extrude "Extrude20" cut sketch "Sketch15" against normal blind 4 contours A0 | A1 picked at (165.390759, -10.692633) picked at (145.390759, -10.692633) bodies 5
sketch "Sketch16" plane through (190.147805, 0, 0) normal (-1, 0, 0) x (0, -1, 0)
  line L0 (68.451903, -2) -> (28.451903, -2)
  line L1 (28.451903, -2) -> (28.451903, -17)
  line L2 (28.451903, -17) -> (68.451903, -17)
  line L3 (68.451903, -17) -> (68.451903, -2)
  line L4 (48.451903, -17) -> (48.451903, -2) construction
  line L5 (48.451903, -17) -> (28.451903, -2) construction
  arc A0 (48.451903, -17) -> (49.022649, -16.239005) centre (48.737276, -16.619502) ccw construction
  line L6 (49.022649, -16.239005) -> (68.451903, -2) construction
  circle A1 centre (38.451903, -9.5) radius 2
  circle A2 centre (58.737276, -9.119502) radius 2
  dimension "d209" = 4
  dimension "d210" = 4
  constraint tangent L5 A0
  measures "d209" diameter of A1
  measures "d210" diameter of A2
extrude "Extrude21" cut sketch "Sketch16" against normal blind 4 contours A1 | A2 picked at (37.324183, -9.918779) picked at (57.589354, -8.566692) bodies 5